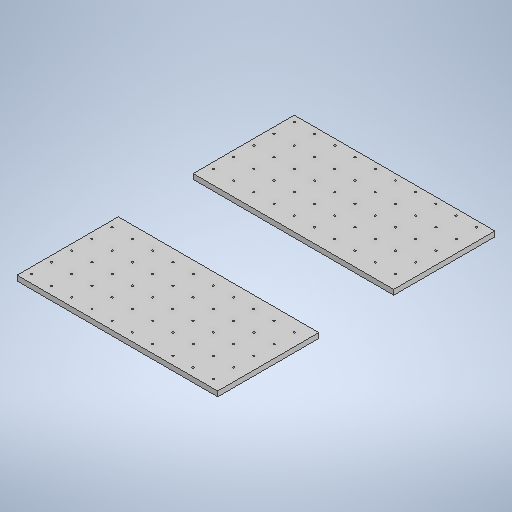
# Autodesk Inventor part: box tray_top
Saved by Autodesk Inventor 2025.3 (Build 293356000, 356)
## iProperties
Created: 2026-02-03
Part Number: box tray_top
Material: Generic
Document SubType Name: Modeling
Designer: AdminForWorker
Density: 1 g/cm^3
Appearance: Default
Title: box tray v1
Author: AdminForWorker
Autodesk Inventor part; units mm, degrees
ref_plane "YZ Plane" through (0, 0, 0) normal (1, 0, 0) x (0, 1, 0)
ref_plane "XZ Plane" through (0, 0, 0) normal (0, 1, 0) x (-1, 0, 0)
ref_plane "XY Plane" through (0, 0, 0) normal (0, 0, 1) x (1, 0, 0)
sketch "Sketch2" plane through (0, 0, 0) normal (0, 1, 0) x (-1, 0, 0)
  line L0 (-476, -174) -> (-476, 174) projected
  line L1 (-924, -174) -> (-476, -174) projected
  line L2 (-924, 174) -> (-924, -174) projected
  line L3 (-476, 174) -> (-924, 174) projected
  point P0 (0, 0)
extrude "Extrusion1" add sketch "Sketch2" along normal blind 6.35
sketch "Sketch3" plane through (0, 6.35, 0) normal (0, 1, 0) x (1, 0, 0)
  circle A0 centre (483.62, 166.38) radius 1.1355
  line L0 (924, 174) -> (476, 174) projected
  line L1 (476, 174) -> (476, -174) projected
  point P0 (0, 0)
  dimension "d8" = 2.271
  dimension "d9" = 7.62
  dimension "d10" = 7.62
  constraints: 1 centre point
  measures "d8" diameter of A0
  measures "d9" distance from line of L0 A0.centre
  measures "d10" distance from line of L1 A0.centre
extrude "Extrusion2" cut sketch "Sketch3" against normal blind 6.35
pattern_linear "Rectangular Pattern1" count 14 spacing 25.4 along (0, 0, 1) count 18 spacing 25.4 along (1, 0, 0) of "Extrusion2"
sketch "Sketch6" plane through (0, 6.35, 0) normal (0, 1, 0) x (1, 0, 0)
  line L0 (476, 174) -> (476, -174) projected
  line L1 (476, 47) -> (727.8243, 47)
  line L2 (727.8243, 47) -> (727.8243, -47)
  line L3 (727.8243, -47) -> (476, -47)
  line L4 (476, -47) -> (476, 47)
  circle A0 centre (485, 0) radius 2.138 projected
  line L5 (924, 174) -> (476, 174) projected
  line L6 (924, 174) -> (727.8243, 174)
  line L7 (727.8243, 174) -> (727.8243, -174)
  line L8 (727.8243, -174) -> (924, -174)
  line L9 (924, -174) -> (924, 174)
  point P0 (0, 0)
  dimension "d29" = 348
  dimension "d33" = 0
  dimension "d37" = 127
  dimension "d38" = 127
  constraints: 16 end point, 4 parallel, 2 horizontal, 2 perpendicular, 1 point on line
  measures "d29" distance of L7.end L6.end
  measures "d33" distance between parallel lines of L2 L7
  measures "d37" distance between parallel lines of L1 L5
  measures "d38" distance of L3.end L0.end
extrude "Extrusion6" cut sketch "Sketch6" against normal blind 6.35 contours L1 L2 L3 L0 | L5 L9 L8 L7 L2 | A0
body "Solid2"
